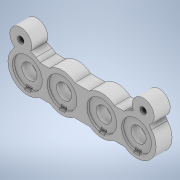
# Autodesk Inventor part: switch_mount_2
Saved by Autodesk Inventor 2022.2 (Build 262287000, 287)
## iProperties
Created: 2022-01-27
Part Number: switch_mount_2
Material: Generic
Document SubType Name: Modeling
Designer: hugof
Density: 1 g/cm^3
Appearance: Default
Author: hugof
Autodesk Inventor part; units mm, degrees
ref_plane "YZ Plane" through (0, 0, 0) normal (1, 0, 0) x (0, 1, 0)
ref_plane "XZ Plane" through (0, 0, 0) normal (0, 1, 0) x (-1, 0, 0)
ref_plane "XY Plane" through (0, 0, 0) normal (0, 0, 1) x (1, 0, 0)
sketch "Sketch2" plane through (0, 0, 0) normal (0, 0, 1) x (1, 0, 0)
  circle A0 centre (0, 0) radius 5.95
  line L0 (0, 0) -> (-4.55, 0)
  line L1 (0, 0) -> (4.55, 0)
  line L2 (0, 0) -> (0, 4.55)
  line L3 (0, 0) -> (0, -4.55)
  line L4 (-4.55, 0) -> (-4.55, -1.8847)
  line L5 (0, 0) -> (2.5958, -2.5958)
  line L6 (0, 0) -> (3.671, 0) construction
  line L7 (3.2173, -3.2173) -> (-3.2173, 3.2173)
  line L8 (0, 0) -> (-3.2173, -3.2173)
  line L9 (0, 0) -> (3.2173, 3.2173)
  line L10 (-3.2173, -3.2173) -> (-1.8847, -4.55)
  line L11 (-3.2173, -3.2173) -> (-4.55, -1.8847)
  line L12 (3.2173, -3.2173) -> (1.8847, -4.55)
  line L13 (3.2173, -3.2173) -> (4.55, -1.8847)
  line L14 (4.55, 0) -> (4.55, -1.8847)
  line L15 (4.55, 0) -> (4.55, 1.8847)
  line L16 (3.2173, 3.2173) -> (4.55, 1.8847)
  line L17 (3.2173, 3.2173) -> (1.8847, 4.55)
  line L18 (0, 4.55) -> (1.8847, 4.55)
  line L19 (0, 4.55) -> (-1.8847, 4.55)
  line L20 (-3.2173, 3.2173) -> (-1.8847, 4.55)
  line L21 (-3.2173, 3.2173) -> (-4.55, 1.8847)
  line L22 (0, -4.55) -> (1.8847, -4.55)
  line L23 (0, -4.55) -> (-1.8847, -4.55)
  line L24 (-4.55, 0) -> (-4.55, 1.8847)
  line L25 (5.95, 0) -> (7.95, 0)
  circle A1 centre (13.9, 0) radius 5.95
  line L26 (6.95, 0) -> (6.95, 2.7112)
  line L27 (-7.95, 7.8017) -> (51.65, 7.8017)
  line L28 (18.45, 0) -> (18.45, 1.8847)
  line L29 (18.45, 0) -> (18.45, -1.8847)
  line L30 (13.9, 0) -> (18.45, 0)
  line L31 (13.9, 0) -> (13.9, 4.55)
  line L32 (13.9, 0) -> (13.9, -4.55)
  line L33 (13.9, -4.55) -> (15.7847, -4.55)
  line L34 (13.9, 4.55) -> (12.0153, 4.55)
  line L35 (13.9, 0) -> (10.6827, 3.2173)
  line L36 (13.9, 0) -> (11.3042, -2.5958)
  line L37 (13.9, -4.55) -> (12.0153, -4.55)
  line L38 (10.6827, 3.2173) -> (9.35, 1.8847)
  line L39 (9.35, 0) -> (9.35, -1.8847)
  line L40 (10.6827, -3.2173) -> (17.1173, 3.2173)
  line L41 (10.6827, -3.2173) -> (9.35, -1.8847)
  circle A2 centre (13.9, 0) radius 5.95
  line L42 (10.6827, -3.2173) -> (12.0153, -4.55)
  line L43 (13.9, 0) -> (9.35, 0)
  line L44 (9.35, 0) -> (9.35, 1.8847)
  line L45 (13.9, 0) -> (10.229, 0) construction
  line L46 (17.1173, 3.2173) -> (15.7847, 4.55)
  line L47 (10.6827, 3.2173) -> (12.0153, 4.55)
  line L48 (13.9, 4.55) -> (15.7847, 4.55)
  line L49 (17.1173, 3.2173) -> (18.45, 1.8847)
  line L50 (17.1173, -3.2173) -> (18.45, -1.8847)
  line L51 (17.1173, -3.2173) -> (15.7847, -4.55)
  line L52 (13.9, 0) -> (17.1173, -3.2173)
  line L53 (21.85, 7.8017) -> (21.85, -7.8017)
  line L54 (51.65, -7.8017) -> (-7.95, -7.8017)
  line L55 (43.7, -4.55) -> (41.8153, -4.55)
  line L56 (43.7, 4.55) -> (41.8153, 4.55)
  line L57 (40.4827, 3.2173) -> (41.8153, 4.55)
  line L58 (43.7, 0) -> (41.1042, -2.5958)
  line L59 (43.7, 0) -> (40.029, 0) construction
  line L60 (43.7, 0) -> (39.15, 0)
  line L61 (40.4827, -3.2173) -> (39.15, -1.8847)
  line L62 (40.4827, 3.2173) -> (39.15, 1.8847)
  line L63 (39.15, 0) -> (39.15, -1.8847)
  line L64 (37.75, 0) -> (35.75, 0)
  line L65 (36.75, 0) -> (36.75, 2.7112)
  line L66 (39.15, 0) -> (39.15, 1.8847)
  line L67 (40.4827, -3.2173) -> (46.9173, 3.2173)
  line L68 (43.7, 0) -> (43.7, 4.55)
  line L69 (43.7, 0) -> (43.7, -4.55)
  line L70 (43.7, -4.55) -> (45.5847, -4.55)
  line L71 (43.7, 4.55) -> (45.5847, 4.55)
  line L72 (43.7, 0) -> (48.25, 0)
  line L73 (48.25, 0) -> (48.25, -1.8847)
  line L74 (46.9173, -3.2173) -> (48.25, -1.8847)
  line L75 (43.7, 0) -> (40.4827, 3.2173)
  circle A3 centre (43.7, 0) radius 5.95
  line L76 (40.4827, -3.2173) -> (41.8153, -4.55)
  line L77 (43.7, 0) -> (46.9173, -3.2173)
  line L78 (46.9173, -3.2173) -> (45.5847, -4.55)
  line L79 (46.9173, 3.2173) -> (45.5847, 4.55)
  line L80 (48.25, 0) -> (48.25, 1.8847)
  line L81 (46.9173, 3.2173) -> (48.25, 1.8847)
  line L82 (33.0173, -3.2173) -> (31.6847, -4.55)
  line L83 (29.8, 0) -> (33.471, 0) construction
  line L84 (29.8, 0) -> (34.35, 0)
  line L85 (29.8, 0) -> (32.3958, -2.5958)
  line L86 (29.8, -4.55) -> (31.6847, -4.55)
  line L87 (29.8, 0) -> (29.8, -4.55)
  line L88 (29.8, 4.55) -> (31.6847, 4.55)
  line L89 (29.8, 0) -> (29.8, 4.55)
  line L90 (29.8, -4.55) -> (27.9153, -4.55)
  line L91 (29.8, 0) -> (26.5827, -3.2173)
  line L92 (26.5827, -3.2173) -> (27.9153, -4.55)
  line L93 (26.5827, 3.2173) -> (27.9153, 4.55)
  line L94 (29.8, 0) -> (25.25, 0)
  line L95 (33.0173, -3.2173) -> (26.5827, 3.2173)
  circle A4 centre (29.8, 0) radius 5.95
  circle A5 centre (29.8, 0) radius 5.95
  line L96 (25.25, 0) -> (25.25, -1.8847)
  line L97 (25.25, 0) -> (25.25, 1.8847)
  line L98 (26.5827, 3.2173) -> (25.25, 1.8847)
  line L99 (26.5827, -3.2173) -> (25.25, -1.8847)
  line L100 (33.0173, -3.2173) -> (34.35, -1.8847)
  line L101 (33.0173, 3.2173) -> (34.35, 1.8847)
  line L102 (29.8, 4.55) -> (27.9153, 4.55)
  line L103 (29.8, 0) -> (33.0173, 3.2173)
  line L104 (33.0173, 3.2173) -> (31.6847, 4.55)
  line L105 (34.35, 0) -> (34.35, 1.8847)
  line L106 (34.35, 0) -> (34.35, -1.8847)
  line L107 (-7.95, 7.8017) -> (-7.95, -7.8017)
  line L108 (51.65, -7.8017) -> (51.65, 7.8017)
  dimension "d0" = 4.55
  dimension "d1" = 4.55
  dimension "d2" = 4.55
  dimension "d3" = 4.55
  dimension "d4" = 45
  constraints: 218 end point, 65 symmetric about line, 10 vertical, 9 perpendicular, 7 horizontal, 7 midpoint, 6 horizontal alignment, 4 coincident, 1 equal length, 1 parallel, 12 other
  measures "d0" distance of L0.start L0.end
  measures "d1" distance of L0.start L1.end
  measures "d2" distance of L0.start L2.end
  measures "d3" distance of L0.start L3.end
  measures "d4" angle of L5 L6
extrude "Extrusion1" add sketch "Sketch2" along normal blind 1.6 contours A0 | A1 | L27 L53 L54 L107 | L27 L108 L54 L53 | A3 | A4
sketch "Sketch3" plane through (0, 0, 1.6) normal (0, 0, 1) x (1, 0, 0)
  circle A0 centre (0, 0) radius 3.05
  line L0 (-7.95, -7.8017) -> (51.65, -7.8017) projected
  line L1 (51.65, -7.8017) -> (51.65, 7.8017) projected
  line L2 (51.65, 7.8017) -> (-7.95, 7.8017) projected
  line L3 (-7.95, 7.8017) -> (-7.95, -7.8017) projected
  line L4 (-4.55, 1.8847) -> (-1.8847, 4.55) projected
  line L5 (-1.8847, 4.55) -> (1.8847, 4.55) projected
  line L6 (1.8847, 4.55) -> (4.55, 1.8847) projected
  line L7 (4.55, 1.8847) -> (4.55, -1.8847) projected
  line L8 (4.55, -1.8847) -> (1.8847, -4.55) projected
  line L9 (1.8847, -4.55) -> (-1.8847, -4.55) projected
  line L10 (-1.8847, -4.55) -> (-4.55, -1.8847) projected
  line L11 (-4.55, -1.8847) -> (-4.55, 1.8847) projected
  line L12 (18.45, -1.8847) -> (15.7847, -4.55) projected
  line L13 (15.7847, -4.55) -> (12.0153, -4.55) projected
  line L14 (12.0153, -4.55) -> (9.35, -1.8847) projected
  line L15 (9.35, -1.8847) -> (9.35, 1.8847) projected
  line L16 (9.35, 1.8847) -> (12.0153, 4.55) projected
  line L17 (12.0153, 4.55) -> (15.7847, 4.55) projected
  line L18 (15.7847, 4.55) -> (18.45, 1.8847) projected
  line L19 (18.45, 1.8847) -> (18.45, -1.8847) projected
  line L20 (48.25, -1.8847) -> (45.5847, -4.55) projected
  line L21 (45.5847, -4.55) -> (41.8153, -4.55) projected
  line L22 (41.8153, -4.55) -> (39.15, -1.8847) projected
  line L23 (39.15, -1.8847) -> (39.15, 1.8847) projected
  line L24 (39.15, 1.8847) -> (41.8153, 4.55) projected
  line L25 (41.8153, 4.55) -> (45.5847, 4.55) projected
  line L26 (45.5847, 4.55) -> (48.25, 1.8847) projected
  line L27 (48.25, 1.8847) -> (48.25, -1.8847) projected
  line L28 (34.35, 1.8847) -> (34.35, -1.8847) projected
  line L29 (34.35, -1.8847) -> (31.6847, -4.55) projected
  line L30 (31.6847, -4.55) -> (27.9153, -4.55) projected
  line L31 (27.9153, -4.55) -> (25.25, -1.8847) projected
  line L32 (25.25, -1.8847) -> (25.25, 1.8847) projected
  line L33 (25.25, 1.8847) -> (27.9153, 4.55) projected
  line L34 (27.9153, 4.55) -> (31.6847, 4.55) projected
  line L35 (31.6847, 4.55) -> (34.35, 1.8847) projected
  circle A1 centre (13.9, 0) radius 3.05
  circle A2 centre (29.8, 0) radius 3.05
  circle A3 centre (43.7, 0) radius 3.05
  line L36 (9.35, -1.8847) -> (9.35, 1.8847) projected
  line L37 (9.35, 0) -> (10.85, 0)
  line L38 (18.45, 1.8847) -> (18.45, -1.8847) projected
  line L39 (18.45, 0) -> (16.95, 0)
  line L40 (25.25, -1.8847) -> (25.25, 1.8847) projected
  line L41 (25.25, 0) -> (26.75, 0)
  line L42 (34.35, 1.8847) -> (34.35, -1.8847) projected
  line L43 (34.35, 0) -> (32.85, 0)
  line L44 (39.15, -1.8847) -> (39.15, 1.8847) projected
  line L45 (39.15, 0) -> (40.65, 0)
  line L46 (46.75, 0) -> (48.25, 0)
  line L47 (48.25, 1.8847) -> (48.25, -1.8847) projected
  line L48 (3.05, 0) -> (4.55, 0)
  line L49 (4.55, 1.8847) -> (4.55, -1.8847) projected
  line L50 (-4.55, -1.8847) -> (-4.55, 1.8847) projected
  line L51 (-4.55, 0) -> (-3.05, 0)
  dimension "d7" = 6.1
  dimension "d8" = 6.1
  dimension "d9" = 6.1
  dimension "d10" = 6.1
  constraints: 16 end point, 8 midpoint, 8 point on circle, 7 point on line, 4 centre point, 1 coincident, 1 perpendicular
  measures "d7" diameter of A0
  measures "d8" diameter of A1
  measures "d9" diameter of A2
  measures "d10" diameter of A3
extrude "Extrusion2" add sketch "Sketch3" along normal blind 4 contours L48 L7 L8 L9 L10 L11 L51 A0 | A0 L51 L11 L4 L5 L6 L7 L48 | L3 L2 L1 L0 | L12 L13 L14 L15 L37 A1 L39 L19 | L39 A1 L37 L15 L16 L17 L18 L19 | L20 L21 L22 L23 L45 A3 L46 L27 | L46 A3 L45 L23 L24 L25 L26 L27 | L28 L43 A2 L41 L32 L33 L34 L35 | L28 L29 L30 L31 L32 L41 A2 L43
sketch "Sketch4" plane through (0, 0, 5.6) normal (0, 0, 1) x (1, 0, 0)
  line L0 (51.65, -7.8017) -> (21.85, -7.8017)
  line L1 (51.65, 7.8017) -> (51.65, -7.8017)
  circle A0 centre (43.7, 0) radius 5.95
  circle A1 centre (29.8, 0) radius 5.95
  line L2 (21.85, 7.8017) -> (21.85, -7.8017)
  line L3 (21.85, 7.8017) -> (51.65, 7.8017)
  line L4 (21.85, -7.8017) -> (-8.35, -7.8017)
  line L5 (29.8, 0) -> (29.8, 7.8017)
  line L6 (29.8, 0) -> (29.8, -7.8017)
  line L7 (43.7, 0) -> (43.7, -7.8017)
  line L8 (43.7, 0) -> (43.7, 7.8017)
  line L9 (-7.95, -7.8017) -> (21.85, -7.8017)
  line L10 (-7.95, 7.8017) -> (-7.95, -7.8017)
  circle A2 centre (0, 0) radius 5.95
  circle A3 centre (13.9, 0) radius 5.95
  line L11 (21.85, 7.8017) -> (-7.95, 7.8017)
  line L12 (13.9, 0) -> (13.9, 7.8017)
  line L13 (13.9, 0) -> (13.9, -7.8017)
  line L14 (0, 0) -> (0, -7.8017)
  line L15 (0, 0) -> (0, 7.8017)
  line L16 (43.7, 0) -> (43.7, -6.35)
  line L17 (43.7, -5.95) -> (43.7, -6.35)
  line L18 (43.7, -6.35) -> (44.8, -6.35)
  line L19 (43.7, -6.35) -> (42.6, -6.35)
  line L20 (44.8, -6.35) -> (44.8, -5.8474)
  line L21 (42.6, -6.35) -> (42.6, -5.8474)
  line L22 (29.8, -5.95) -> (29.8, -6.35)
  line L23 (29.8, -6.35) -> (30.9, -6.35)
  line L24 (29.8, -6.35) -> (28.7, -6.35)
  line L25 (30.9, -6.35) -> (30.9, -5.8474)
  line L26 (28.7, -6.35) -> (28.7, -5.8474)
  line L27 (13.9, -5.95) -> (13.9, -6.35)
  line L28 (13.9, -6.35) -> (15, -6.35)
  line L29 (13.9, -6.35) -> (12.8, -6.35)
  line L30 (15, -6.35) -> (15, -5.8474)
  line L31 (12.8, -6.35) -> (12.8, -5.8474)
  line L32 (0, -5.95) -> (0, -6.35)
  line L33 (0, -6.35) -> (1.1, -6.35)
  line L34 (0, -6.35) -> (-1.1, -6.35)
  line L35 (1.1, -6.35) -> (1.1, -5.8474)
  line L36 (-1.1, -6.35) -> (-1.1, -5.8474)
  point P0 (0, 0)
  point P1 (51.65, 0)
  point P2 (-7.95, 0)
  point P3 (-59.6, 0)
  dimension "d13" = 11.9
  dimension "d14" = 11.9
  dimension "d15" = 7.95
  dimension "d16" = 13.9
  dimension "d17" = 7.95
  dimension "d22" = 0.4
  dimension "d23" = 1.1
  dimension "d24" = 1.1
  dimension "d25" = 0.4
  dimension "d26" = 1.1
  dimension "d27" = 1.1
  dimension "d28" = 0.4
  dimension "d29" = 1.1
  dimension "d30" = 1.1
  dimension "d31" = 0.4
  dimension "d32" = 1.1
  dimension "d33" = 1.1
  constraints: 74 end point, 14 point on line, 10 horizontal, 9 symmetric about line, 4 centre point, 4 perpendicular, 4 vertical, 3 collinear, 3 parallel, 3 point on circle, 1 midpoint, 2 other
  measures "d13" diameter of A0
  measures "d14" diameter of A1
  measures "d15" distance from line of L2 L5.start
  measures "d16" distance of L7.start L5.start
  measures "d17" distance from line of L1 L7.start
  measures "d22" distance of L17.start L16.end
  measures "d23" distance of L16.end L18.end
  measures "d24" distance of L16.end L19.end
  measures "d25" distance of L22.start L23.start
  measures "d26" distance of L23.start L25.start
  measures "d27" distance of L23.start L24.end
  measures "d28" distance of L27.start L28.start
  measures "d29" distance of L28.start L30.start
  measures "d30" distance of L28.start L29.end
  measures "d31" distance of L32.start L33.start
  measures "d32" distance of L33.start L35.start
  measures "d33" distance of L33.start L34.end
extrude "Extrusion4" add sketch "Sketch4" along normal blind 0.8 contours L0 L7 L18 L20 A0 L8 L3 L1 | L0 L6 L23 L25 A1 L5 L3 L8 A0 L21 L19 L7 | L0 L2 L3 L5 A1 L26 L24 L6 | L4 L13 L28 L30 A3 L12 L11 L2 | L4 L14 L33 L35 A2 L15 L11 L12 A3 L31 L29 L13 | L4 L10 L11 L15 A2 L36 L34 L14
extrude "Extrusion5" cut sketch "Sketch4" against normal blind 0.8 contours L19 L21 A0 L7 | L7 A0 L20 L18 | L24 L26 A1 L6 | L6 A1 L25 L23 | L29 L31 A3 L13 | L13 A3 L30 L28 | L34 L36 A2 L14 | L14 A2 L35 L33
fillet "Fillet3" radius 1 4 edges at (29.8, -5.95, 5.6) (43.7, -5.95, 5.6) (13.9, -5.95, 5.6) (0, -5.95, 5.6)
sketch "Sketch5" plane through (0, 0, 6.4) normal (0, 0, 1) x (1, 0, 0)
  arc A0 (15, -5.8474) -> (12.8, -5.8474) centre (13.9, 0) ccw projected
  line L0 (51.65, 7.8017) -> (-7.95, 7.8017) projected
  arc A1 (1.1, -5.8474) -> (-1.1, -5.8474) centre (0, 0) ccw projected
  circle A2 centre (0, 0) radius 7.8017
  circle A3 centre (13.9, 0) radius 7.8017
  circle A4 centre (29.8, 0) radius 3.05 projected
  circle A5 centre (29.8, 0) radius 7.8017
  circle A6 centre (43.7, 0) radius 3.05 projected
  circle A7 centre (43.7, 0) radius 7.8017
  line L1 (0, 7.8017) -> (13.9, 7.8017)
  line L2 (29.8, 7.8017) -> (43.7, 7.8017)
  line L3 (-7.95, -7.8017) -> (51.65, -7.8017) projected
  line L4 (29.8, -7.8017) -> (43.7, -7.8017)
  line L5 (13.9, -7.8017) -> (0, -7.8017)
  line L6 (51.65, 7.8017) -> (-7.95, 7.8017) projected
  line L7 (0, 7.8017) -> (-7.95, 7.8017)
  line L8 (-7.95, 7.8017) -> (-7.95, -7.8017) projected
  line L9 (-7.95, 7.8017) -> (-7.95, -7.8017)
  line L10 (-7.95, -7.8017) -> (0, -7.8017)
  line L11 (51.65, -7.8017) -> (51.65, 7.8017) projected
  line L12 (43.7, 7.8017) -> (51.65, 7.8017)
  line L13 (51.65, 7.8017) -> (51.65, -7.8017)
  line L14 (51.65, -7.8017) -> (43.7, -7.8017)
  line L15 (5.0462, 5.95) -> (8.8538, 5.95)
  line L16 (18.9462, 5.95) -> (24.7538, 5.95)
  line L17 (34.8462, 5.95) -> (38.6538, 5.95)
  line L18 (39, -6.2271) -> (34.5, -6.2271)
  line L19 (25.1, -6.2271) -> (18.6, -6.2271)
  line L20 (9.2, -6.2271) -> (4.7, -6.2271)
  point P0 (0, 0)
  point P1 (49.15, 7.8017)
  point P2 (-5.45, 7.8017)
  point P3 (-5.45, -7.8017)
  point P4 (49.15, -7.8017)
  point P5 (13.9, -7.8017)
  point P6 (0, -7.8017)
  constraints: 32 end point, 20 point on circle, 14 point on line, 4 centre point, 4 coincident, 4 tangent, 3 horizontal, 3 perpendicular, 2 collinear, 1 parallel
extrude "Extrusion6" cut sketch "Sketch5" against normal through all contours L11 L3 A7 L0 | A7 L17 A5 L0 | A5 L16 A3 L0 | L3 A5 L18 A7 | A3 L15 A2 L0 | L3 A3 L19 A5 | A2 L3 L8 L0 | L3 A2 L20 A3
sketch "Sketch6" plane through (0, 0, 6.4) normal (0, 0, 1) x (1, 0, 0)
  circle A0 centre (43.7, 0) radius 3.05 projected
  circle A1 centre (0, 0) radius 3.05 projected
  circle A2 centre (46.35, 10) radius 1.3
  circle A3 centre (-2.65, 10) radius 1.3
  line L0 (46.35, 10) -> (43.7, 10)
  line L1 (43.7, 0) -> (43.7, 10)
  line L2 (0, 0) -> (0, 10)
  line L3 (0, 10) -> (-2.65, 10)
  line L4 (43.7, 10) -> (0, 10)
  circle A4 centre (46.35, 10) radius 4.3952
  arc A5 (44.8, -5.8474) -> (42.6, -5.8474) centre (43.7, 0) ccw projected
  circle A6 centre (-2.65, 10) radius 4.3952
  arc A7 (1.1, -5.8474) -> (-1.1, -5.8474) centre (0, 0) ccw projected
  line L5 (46.35, 10) -> (40.2546, 6.9997)
  arc A8 (39, -6.2271) -> (38.6538, 5.95) centre (43.7, 0) ccw projected
  line L6 (46.35, 10) -> (49.6889, 5)
  arc A9 (5.0462, 5.95) -> (4.7, -6.2271) centre (0, 0) ccw projected
  line L7 (-2.65, 10) -> (3.4454, 6.9997)
  line L8 (-2.65, 10) -> (-5.9889, 5)
  point P0 (1.2934, 8.059)
  point P1 (-5.0908, 6.3449)
  point P2 (42.4066, 8.059)
  point P3 (48.7908, 6.3449)
  dimension "d42" = 49
  dimension "d43" = 2.6
  dimension "d44" = 2.6
  constraints: 18 end point, 6 perpendicular, 4 centre point, 4 point on circle, 3 horizontal, 3 tangent, 2 coincident, 1 collinear
  measures "d42" distance of L0.start L3.end
  measures "d43" diameter of A2
  measures "d44" diameter of A3
extrude "Extrusion7" add sketch "Sketch6" against normal up to surface (6.4 mm away) contours A2 L0 L4 A4 L6 | A2 L5 L1 L0 | L6 A4 A8 L1 L5 A2 | L1 L5 A4 L4 | L6 A8 A4 | L1 A8 A4 L5 | A4 A8 L5 | L3 L2 L7 A3 | A3 L8 A6 L4 L3 | A3 L7 L2 A9 A6 L8 | L4 A6 L7 L2 | A6 A9 L8 | L7 A6 A9 L2 | L7 A9 A6
body "Solid1"
